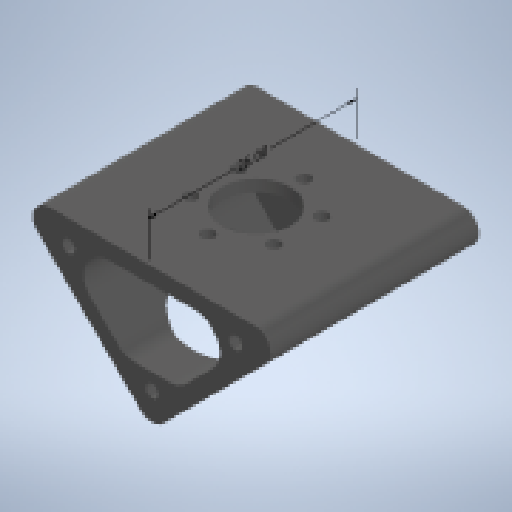
# Autodesk Inventor part: hipjoint_middle
Saved by Autodesk Inventor 2024.1 (Build 281209000, 209)
## iProperties
Created: 2024-02-13
Part Number: hipjoint_middle
Material: 一般
Document SubType Name: Modeling
Designer: hibik
Density: 1 g/cm^3
Appearance: 既定
Author: hibik
Autodesk Inventor part; units mm, degrees
ref_plane "YZ Plane" through (0, 0, 0) normal (1, 0, 0) x (0, 1, 0)
ref_plane "XZ Plane" through (0, 0, 0) normal (0, 1, 0) x (-1, 0, 0)
ref_plane "XY Plane" through (0, 0, 0) normal (0, 0, 1) x (1, 0, 0)
sketch "スケッチ1" plane through (0, 0, 0) normal (0, 0, 1) x (1, 0, 0)
  line L0 (0, 0) -> (-17.6777, 17.6777)
  line L1 (-17.6777, 17.6777) -> (17.6777, 17.6777)
  line L2 (17.6777, 17.6777) -> (0, 0)
  line L3 (-17.6777, 17.6777) -> (-21.2487, 14.1066)
  line L4 (0, 0) -> (-2.2909, -2.2909)
  circle A0 centre (-10.435, 14.6777) radius 0.8
  circle A1 centre (10.435, 14.6777) radius 0.8
  circle A2 centre (0, 4.2426) radius 0.8
  dimension "d0" = 25
  dimension "d1" = 45
  dimension "d5" = 1.6
  dimension "d6" = 1.6
  dimension "d7" = 1.6
  dimension "d8" = 3
  dimension "d9" = 3
  dimension "d10" = 3
  dimension "d11" = 3
  dimension "d12" = 3
  dimension "d13" = 3
  constraints: 10 end point, 3 centre point, 3 perpendicular, 1 horizontal
  measures "d0" distance between parallel lines of L4 L3
  measures "d1" angle of L1 L0
  measures "d5" diameter of A0
  measures "d6" diameter of A1
  measures "d7" diameter of A2
  measures "d8" distance from line of L0 A0.centre
  measures "d9" distance from line of L1 A0.centre
  measures "d10" distance from line of L1 A1.centre
  measures "d11" distance from line of L2 A1.centre
  measures "d12" distance from line of L2 A2.centre
  measures "d13" distance from line of L0 A2.centre
extrude "押し出し1" add sketch "スケッチ1" along normal blind 26
fillet "フィレット1" radius 2 3 edges at (17.6777, 17.6777, 13) (0, 0, 13) (-17.6777, 17.6777, 13)
sketch "スケッチ2" plane through (-12.8492, 17.6777, 0) normal (0, 1, 0) x (1, 0, 0)
  line L0 (0, -26) -> (0, 0) projected
  line L1 (25.6985, -26) -> (0, -26) projected
  line L2 (25.6985, 0) -> (25.6985, -26) projected
  line L3 (25.6985, 0) -> (0, 0) projected
  line L4 (25.6985, -26) -> (0, 0)
  line L5 (0, -26) -> (-2, -26) projected
  line L6 (0, -26) -> (25.6985, 0)
  circle A0 centre (12.8492, -13) radius 4.25
  circle A1 centre (12.8492, -13) radius 6 construction
  circle A2 centre (12.8492, -19) radius 0.8
  circle A3 centre (17.0919, -17.2426) radius 0.8
  circle A4 centre (18.8492, -13) radius 0.8
  circle A5 centre (17.0919, -8.7574) radius 0.8
  circle A6 centre (12.8492, -7) radius 0.8
  circle A7 centre (8.6066, -8.7574) radius 0.8
  circle A8 centre (12.8492, -13) radius 8
  circle A9 centre (6.8492, -13) radius 0.8
  circle A10 centre (8.6066, -17.2426) radius 0.8
  point P0 (12.8492, 0)
  point P1 (-1.4142, -26)
  dimension "d15" = 12
  dimension "d14" = 8.5
  dimension "d16" = 1.6
  dimension "d23" = 360
  dimension "d25" = 16
  constraints: 10 centre point, 4 end point, 2 coincident, 2 midpoint, 2 vertical alignment, 19 other
  measures "d14" diameter of A0
  measures "d16" diameter of A2
  measures "d25" diameter of A8
extrude "押し出し2" cut sketch "スケッチ2" against normal through all contours A8 L4 A7 A0 L6 A10 | L6 A10 A0 L4 A3 A8 | A8 L6 A5 A0 L4 A7 | L4 A3 A0 L6 A5 A8 | A10 L6 | L6 A10 | A7 L4 | L4 A7 | A3 L4 | L4 A3 | A5 L6 | L6 A5 | A0 L4 L6 | L6 L4 A0 | A0 L6 L4 | L4 L6 A0 | A2 | A4 | A6 | A9
extrude "押し出し3" add sketch "スケッチ2" against normal blind 1.5 contours A8 L4 A7 A0 L6 A10 | L6 A10 A0 L4 A3 A8 | A8 L6 A5 A0 L4 A7 | L4 A3 A0 L6 A5 A8
sketch "スケッチ4" plane through (0, 0, 26) normal (0, 0, 1) x (1, 0, 0)
  line L0 (-4.2929, 7.1213) -> (-7.6066, 10.435) projected
  arc A0 (-7.6066, 14.6777) -> (-7.6066, 10.435) centre (-5.4853, 12.5563) ccw projected
  arc A1 (-5.364, 15.6777) -> (-7.4853, 14.799) centre (-5.364, 12.6777) ccw projected
  line L1 (-7.6066, 14.6777) -> (-7.4853, 14.799) projected
  line L2 (-5.364, 15.6777) -> (5.364, 15.6777) projected
  arc A2 (7.4853, 14.799) -> (5.364, 15.6777) centre (5.364, 12.6777) ccw projected
  arc A3 (7.6066, 10.435) -> (7.6066, 14.6777) centre (5.4853, 12.5563) ccw projected
  line L3 (7.4853, 14.799) -> (7.6066, 14.6777) projected
  line L4 (7.6066, 10.435) -> (4.2929, 7.1213) projected
  arc A4 (2.1716, 6.2426) -> (4.2929, 7.1213) centre (2.1716, 9.2426) ccw projected
  line L5 (2.1716, 6.2426) -> (-2.1716, 6.2426) projected
  arc A5 (-4.2929, 7.1213) -> (-2.1716, 6.2426) centre (-2.1716, 9.2426) ccw projected
  point P0 (0, 0)
extrude "押し出し5" cut sketch "スケッチ4" against normal blind 21
equation "\"d9\" = d8"
equation "\"d10\" = d8"
equation "\"d11\" = d8"
equation "\"d12\" = d8"
equation "\"d13\" = d8"
